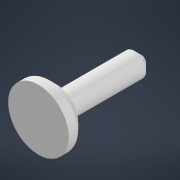
# Autodesk Inventor part: CorePin
Saved by Autodesk Inventor 2021 (Build 250183000, 183)
## iProperties
Created: 2020-06-05
Part Number: CorePin
Material: Generic
Document SubType Name: Modeling
Designer: Shadow
Density: 1 g/cm^3
Appearance: Default
Author: Shadow
## iProperties of the stored document _3DPrint.ipt
Created: 2020-06-05
Part Number: _3DPrint
Material: Generic
Document SubType Name: Modeling
Designer: Shadow
Density: 1 g/cm^3
Appearance: Default
Author: Shadow
Autodesk Inventor part; units mm, degrees
ref_plane "YZ Plane" through (0, 0, 0) normal (1, 0, 0) x (0, 1, 0)
ref_plane "XZ Plane" through (0, 0, 0) normal (0, 1, 0) x (-1, 0, 0)
ref_plane "XY Plane" through (0, 0, 0) normal (0, 0, 1) x (1, 0, 0)
sketch "Sketch1" plane through (0, 0, 0) normal (0, 0, 1) x (1, 0, 0)
  circle A0 centre (13.1805, 11.7967) radius 1.8375 projected
  circle A1 centre (13.1805, 11.7967) radius 1.2375
  point P0 (0, 0)
  dimension "d13" = 0.6
  constraints: 1 centre point, 1 coincident
  measures "d13" radial gap between concentric circles of A1 A0
extrude "Extrusion1" add sketch "Sketch1" against normal blind 9 contours A1
sketch "Sketch2" plane through (13.1805, 11.7967, 0) normal (0, 0, 1) x (1, 0, 0)
  circle A0 centre (0, 0) radius 1.2375 projected
  circle A1 centre (0, 0) radius 3.2375
  point P0 (-13.1805, -11.7967)
  dimension "d3" = 2
  constraints: 1 centre point
  measures "d3" radial gap between concentric circles of A0 A1
extrude "Extrusion2" add sketch "Sketch2" along normal blind 2 contours A0 | A1
chamfer "Chamfer1" distance 1 angle 45 1 edges at (9.943, 11.7967, 0)
fillet "Fillet1" radius 0.5 2 edges at (10.943, 11.7967, 0) (9.943, 11.7967, 1)
chamfer "Chamfer2" distance 0.75 angle 45 1 edges at (11.943, 11.7967, -9)
body "Solid1"
